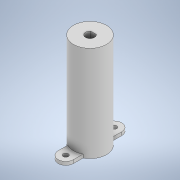
# Autodesk Inventor part: Arm
Saved by Autodesk Inventor 2021 (Build 250183000, 183)
## iProperties
Created: 2024-01-01
Part Number: Arm
Material: Generic
Document SubType Name: Modeling
Designer: brybr
Density: 1 g/cm^3
Appearance: Default
Author: brybr
Autodesk Inventor part; units mm, degrees
ref_plane "YZ Plane" through (0, 0, 0) normal (1, 0, 0) x (0, 1, 0)
ref_plane "XZ Plane" through (0, 0, 0) normal (0, 1, 0) x (-1, 0, 0)
sketch "Sketch1" plane through (0, 0, 0) normal (0, 1, 0) x (-1, 0, 0)
  line L0 (0, 0) -> (4.8, 0) construction
  circle A0 centre (0, 0) radius 2.5 construction
  circle A1 centre (0, 0) radius 2.65
  line L1 (0.0078, 2.5) -> (0.0078, -2.1) construction
  line L2 (0.0078, 2.5) -> (4.6078, 2.5) construction
  line L3 (0.0078, -2.1) -> (1.6163, -2.1)
  line L4 (0.0078, -2.1) -> (-1.6163, -2.1)
  line L5 (0.0078, -2.1) -> (1.6319, -2.1) construction
  circle A2 centre (0, 0) radius 7.5 construction
  circle A3 centre (0, 0) radius 7.7
  circle A4 centre (0, 0) radius 9.7
  dimension "d5" = 5
  dimension "d6" = 0.15
  dimension "d7" = 4.6
  dimension "d8" = 90
  dimension "d9" = 90
  dimension "d10" = 180
  dimension "d26" = 15
  dimension "d27" = 0.2
  dimension "d28" = 2
  constraints: 12 end point, 4 centre point, 3 coincident, 3 horizontal, 2 equal length, 2 point on circle, 1 vertical, 3 other
  measures "d7" distance of L1.start L1.end
  measures "d8" angle of L1 L2
  measures "d9" angle of L3 L1
  measures "d10" angle of L4 L5
  measures "d26" diameter of A2
  measures "d27" radial gap between concentric circles of A2 A3
  measures "d28" radial gap between concentric circles of A3 A4
extrude "Extrusion5" add sketch "Sketch1" along normal blind 16 contours L4 L3 A1 | A3 | A4 picked at (-0.9103, -2.2002)
extrude "Extrusion6" add sketch "Sketch1" along normal blind 1 contours A1 L3 L4 picked at (0.0374, 1.0538)
extrude "Extrusion7" add sketch "Sketch1" against normal blind 40 contours A4
ref_plane "Work Plane1" through (0, 0, -9.7) normal (0, 0, 1) x (1, 0, 0)
sketch "Sketch3" plane through (0, 0, -9.7) normal (0, 0, 1) x (1, 0, 0)
  circle A0 centre (0, 8.5) radius 1.5
  circle A1 centre (0, 8.5) radius 3
  point P0 (0, 0)
  dimension "d35" = 3
  dimension "d36" = 6
  constraints: 2 centre point, 1 coincident
  measures "d35" diameter of A0
  measures "d36" diameter of A1
extrude "Extrusion8" cut sketch "Sketch3" along normal blind 7.7 contours A0
extrude "Extrusion9" cut sketch "Sketch3" along normal blind 10
sketch "Sketch4" plane through (0, -40, 0) normal (0, -1, 0) x (1, 0, 0)
  circle A0 centre (0, 0) radius 9.7 projected
  circle A1 centre (0, 14.2) radius 1.5
  line L0 (0, 12.7) -> (0, 9.7) construction
  circle A2 centre (0, 14.2) radius 4.5
  line L1 (4.5, 14.2) -> (4.5, 8.593)
  line L2 (-4.5, 14.2) -> (-4.5, 8.593)
  circle A3 centre (0, 0) radius 9.7 projected
  dimension "d42" = 3
  dimension "d43" = 3
  dimension "d44" = 3
  constraints: 6 end point, 5 point on circle, 3 tangent, 2 parallel, 2 vertical, 1 centre point, 1 vertical alignment, 2 other
  measures "d43" distance of L0.start L0.end
extrude "Extrusion10" add sketch "Sketch4" against normal blind 2 contours A0 A2 L1 | L2 A2 A0 | A2
pattern_circular "Circular Pattern1" count 2 over 360 about axis through (0, 0, 0) along (0, -1, 0) of "Extrusion10"
body "Solid2"
